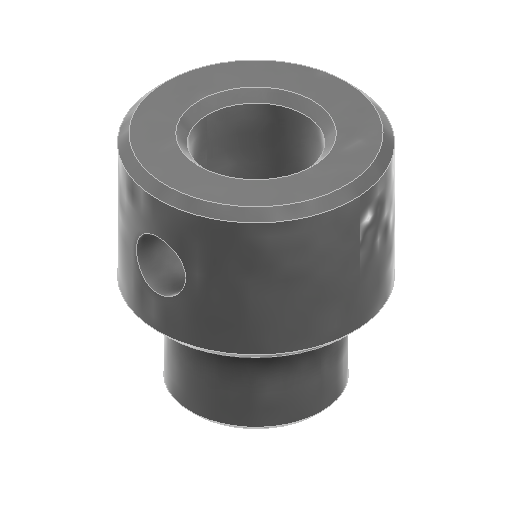
# Autodesk Inventor part: Acople_EJE
Saved by Autodesk Inventor 2025 (Build 290162000, 162)
## iProperties
Created: 2026-02-06
Part Number: Acople_EJE
Material: Plástico ABS
Document SubType Name: Modeling
Designer: HP
Density: 1.06 g/cm^3
Appearance: Negro
Author: HP
Autodesk Inventor part; units mm, degrees
ref_plane "XZ Plane" through (0, 0, 0) normal (0, 1, 0) x (-1, 0, 0)
sketch "Boceto9" plane through (0, 0, 0) normal (0, 1, 0) x (-1, 0, 0)
  circle A0 centre (0, 0) radius 6
  circle A1 centre (0, 0) radius 2.975
  dimension "d34" = 12
  dimension "d35" = 5.95
  constraints: 2 centre point, 2 coincident
  measures "d34" diameter of A0
  measures "d35" diameter of A1
extrude "Extrusión9" add sketch "Boceto9" along normal blind 8
sketch "Boceto10" plane through (0, 0, 0) normal (0, -1, 0) x (1, 0, 0)
  circle A0 centre (0, 0) radius 6 projected
  circle A1 centre (0, 0) radius 2.975 projected
  circle A2 centre (0, 0) radius 5
  dimension "d38" = 1
  constraints: 1 centre point
  measures "d38" radial gap between concentric circles of A0 A2
extrude "Extrusión10" add sketch "Boceto10" along normal blind 5 contours A2
sketch "Boceto11" plane through (0, 0, 0) normal (0, -1, 0) x (1, 0, 0)
  circle A0 centre (0, 0) radius 2.975 projected
extrude "Extrusión11" add sketch "Boceto11" along normal blind 2
sketch "Boceto12" plane through (0, -2, 0) normal (0, -1, 0) x (1, 0, 0)
  circle A0 centre (0, 0) radius 2.5
  circle A1 centre (0, 0) radius 2.975 projected
  dimension "d43" = 5
  constraints: 1 centre point, 1 coincident
  measures "d43" diameter of A0
extrude "Extrusión12" add sketch "Boceto12" along normal blind 3
sketch "Boceto13" plane through (0, -5, 0) normal (0, -1, 0) x (1, 0, 0)
  circle A0 centre (0, 0) radius 4
  circle A1 centre (0, 0) radius 5 projected
  dimension "d46" = 8
  constraints: 1 centre point, 1 coincident
  measures "d46" diameter of A0
extrude "Extrusión13" cut sketch "Boceto13" against normal blind 5
chamfer "Chaflán4" distance 0.25 angle 45 1 edges at (-4, -5, 0)
fillet "Empalme2" radius 0.5 1 edges at (-4, 0, 0)
chamfer "Chaflán5" distance 0.5 angle 45 2 edges at (6, 0, 0) (6, 8, 0)
chamfer "Chaflán6" distance 0.5 angle 45 1 edges at (2.975, 8, 0)
ref_plane "Plano de trabajo3" through (0, 0, 6) normal (0, 0, 1) x (1, 0, 0)
sketch "Boceto14" plane through (0, 0, 6) normal (0, 0, 1) x (1, 0, 0)
  line L0 (-6, 0.5) -> (6, 0.5) projected
  line L1 (6, 7.5) -> (-6, 7.5) projected
  line L2 (0, 0.5) -> (0, 7.5) construction
  circle A0 centre (0, 4) radius 1.5
  point P0 (0, 0)
  dimension "d60" = 3
  constraints: 3 midpoint, 2 end point, 1 centre point
  measures "d60" diameter of A0
extrude "Extrusión14" cut sketch "Boceto14" against normal blind 4
sketch "Boceto1" plane through (0, 0, 0) normal (0, 1, 0) x (-1, 0, 0)
  circle A0 centre (0, 0) radius 15
  dimension "d0" = 30
  constraints: 1 centre point, 1 coincident
  measures "d0" diameter of A0
sketch "Boceto2" plane through (0, 10, 0) normal (0, 1, 0) x (1, 0, 0)
  circle A0 centre (0, 0) radius 2.5
  dimension "d3" = 5
  constraints: 1 centre point, 1 coincident
  measures "d3" diameter of A0
sketch "Boceto3" plane through (0, 0, 0) normal (0, -1, 0) x (1, 0, 0)
  circle A0 centre (0, 0) radius 7.5
  dimension "d6" = 15
  constraints: 1 centre point, 1 coincident
  measures "d6" diameter of A0
sketch "Boceto4" plane through (0, -10, 0) normal (0, -1, 0) x (1, 0, 0)
  circle A0 centre (0, 0) radius 2.975
  dimension "d9" = 5.95
  constraints: 1 centre point, 1 coincident
  measures "d9" diameter of A0
sketch "Boceto6" plane through (0, -10, 0) normal (0, -1, 0) x (1, 0, 0)
  circle A0 centre (0, 0) radius 2.975 projected
  circle A1 centre (0, 0) radius 7.5 projected
sketch "Boceto8" plane through (0, 0, 7.5) normal (0, 0, 1) x (1, 0, 0)
  line L0 (-7.5, -14) -> (7.5, -14) projected
  line L1 (7.5, -2) -> (-7.5, -2) projected
  line L2 (7.5, -2) -> (7.5, -14) projected
  line L3 (-7.5, -2) -> (-7.5, -14) projected
  line L4 (7.5, -8) -> (-7.5, -8) construction
  circle A0 centre (0, -8) radius 1.5
  point P0 (0, 0)
  dimension "d31" = 3
  constraints: 3 midpoint, 2 end point, 1 centre point
  measures "d31" diameter of A0
sketch "Boceto7" plane through (15, 0, 0) normal (1, 0, 0) x (0, 1, 0)
  line L0 (1, 15) -> (1, -15) projected
  line L1 (14, -15) -> (14, 15) projected
  line L2 (1, -15) -> (10, -15) projected
  line L3 (1, 15) -> (10, 15) projected
  line L4 (7.5, 15) -> (7.5, -15) construction
  circle A0 centre (7.5, 0) radius 1.5
  point P0 (0, 0)
  dimension "d27" = 3
  constraints: 2 end point, 2 point on line, 1 centre point, 1 midpoint, 1 other
  measures "d27" diameter of A0
